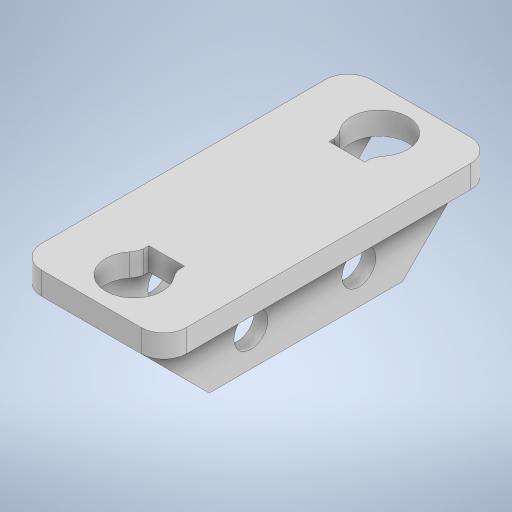
# Autodesk Inventor part: Magnet Mount
Saved by Autodesk Inventor 2023.1 (Build 271208000, 208)
## iProperties
Created: 2022-11-07
Part Number: Magnet Mount
Material: Generic
Document SubType Name: Modeling
Designer: nicol
Density: 1 g/cm^3
Appearance: Default
Author: nicol
Autodesk Inventor part; units mm, degrees
ref_plane "YZ Plane" through (0, 0, 0) normal (1, 0, 0) x (0, 1, 0)
ref_plane "XZ Plane" through (0, 0, 0) normal (0, 1, 0) x (-1, 0, 0)
ref_plane "XY Plane" through (0, 0, 0) normal (0, 0, 1) x (1, 0, 0)
sketch "Sketch1" plane through (0, 0, 0) normal (0, 1, 0) x (-1, 0, 0)
  line L0 (0, 0) -> (6.38, 0)
  line L1 (6.38, 0) -> (6.38, -20.1)
  line L2 (6.38, -20.1) -> (0, -20.1)
  line L3 (0, -20.1) -> (0, 0)
  line L4 (4.68, -1.7) -> (1.56, -1.7)
  line L5 (1.56, -1.7) -> (1.56, -2.17)
  line L6 (1.56, -2.17) -> (4.68, -2.17)
  line L7 (4.68, -2.17) -> (4.68, -1.7)
  line L8 (4.68, -18.03) -> (1.56, -18.03)
  line L9 (1.56, -18.03) -> (1.56, -18.5)
  line L10 (1.56, -18.5) -> (4.68, -18.5)
  line L11 (4.68, -18.5) -> (4.68, -18.03)
  line L12 (7.58, 4.4) -> (-1.2, 4.4)
  line L13 (-1.2, 4.4) -> (-1.2, -24.6)
  line L14 (-1.2, -24.6) -> (7.58, -24.6)
  line L15 (7.58, -24.6) -> (7.58, 4.4)
  circle A0 centre (3.12, -20.9) radius 2.5
  circle A1 centre (3.12, 0.7) radius 2.5
  line L16 (5.105, 3.2) -> (1.56, 3.2) construction
  line L17 (5.6212, -23.4) -> (1.5588, -23.4) construction
  point P0 (3.12, -18.5)
  point P1 (3.82, -1.7)
  point P2 (2.42, -18.5)
  point P3 (2.42, -1.7)
  point P4 (3.82, -18.5)
  dimension "d0" = 20.1
  dimension "d1" = 6.38
  dimension "d2" = 0.47
  dimension "d3" = 3.12
  dimension "d4" = 1.7
  dimension "d5" = 1.7
  dimension "d6" = 1.6
  dimension "d7" = 1.7
  dimension "d8" = 5
  dimension "d9" = 1.2
  dimension "d10" = 1.2
  dimension "d11" = 1.2
  dimension "d12" = 1.2
  dimension "d15" = 2.4
  dimension "d16" = 2.4
  constraints: 36 end point, 8 parallel, 6 horizontal, 4 perpendicular, 2 centre point, 2 equal length, 2 tangent, 2 vertical alignment, 1 equal radius, 1 midpoint
  measures "d0" distance of L0.end L1.end
  measures "d1" distance of L0.start L0.end
  measures "d2" distance of L6.end L4.start
  measures "d3" distance of L5.end L6.end
  measures "d4" distance between parallel lines of L1 L7
  measures "d5" distance between parallel lines of L0 L4
  measures "d6" distance between parallel lines of L2 L10
  measures "d7" distance between parallel lines of L1 L11
  measures "d8" diameter of A0
  measures "d9" distance between parallel lines of L13 L3
  measures "d10" distance between parallel lines of L15 L1
  measures "d11" distance between parallel lines of L12 L16
  measures "d12" distance between parallel lines of L14 L17
  measures "d15" distance from line of A0.centre L10
  measures "d16" distance from line of L4 A1.centre
extrude "Extrusion1" add sketch "Sketch1" along normal blind 2 contours L0 A1 L4 L5 L6 L7 L1 L2 A0 L10 L11 L8 L9 L3 | L15 L14 L13 L12
fillet "Fillet1" radius 2 4 edges at (-3.82, 1, -1.7) (-2.42, 1, -1.7) (-2.42, 1, -18.5) (-3.82, 1, -18.5)
sketch "Sketch2" plane through (0, 0, 0) normal (0, -1, 0) x (1, 0, 0)
  line L0 (1.2, 4.4) -> (1.2, -24.6) projected
  line L1 (1.2, 4.4) -> (0, 4.4)
  line L2 (0, 4.4) -> (0, -24.6)
  line L3 (0, -24.6) -> (1.2, -24.6)
  line L4 (1.2, -24.6) -> (1.2, 4.4)
  line L5 (1.2, -24.6) -> (-7.58, -24.6) projected
  line L6 (-7.58, -24.6) -> (-7.58, 4.4) projected
  line L7 (-7.58, 4.4) -> (-6.38, 4.4)
  line L8 (-6.38, 4.4) -> (-6.38, -24.6)
  line L9 (-6.38, -24.6) -> (-7.58, -24.6)
  line L10 (-7.58, -24.6) -> (-7.58, 4.4)
  point P0 (0, 0)
  dimension "d18" = 1.2
  dimension "d19" = 1.2
  constraints: 16 end point, 4 parallel, 2 collinear, 2 horizontal, 2 perpendicular
  measures "d18" distance between parallel lines of L0 L2
  measures "d19" distance of L8.end L9.end
extrude "Extrusion2" add sketch "Sketch2" along normal blind 6
sketch "Sketch3" plane through (1.2, 2, -24.6) normal (0, 0, -1) x (-1, 0, 0)
  line L0 (1.2, -2) -> (7.58, -2) projected
  line L1 (7.58, -2) -> (7.58, -8) projected
  line L2 (8.78, -8) -> (7.58, -8) projected
  line L3 (8.78, -8) -> (8.78, 0) projected
  line L4 (0, 0) -> (8.78, 0) projected
  line L5 (0, -8) -> (0, 0) projected
  line L6 (1.2, -8) -> (0, -8) projected
  line L7 (1.2, -2) -> (1.2, -8) projected
  line L8 (-2, -2) -> (10.78, -2)
  line L9 (10.78, -2) -> (10.78, 0)
  line L10 (10.78, 0) -> (-2, 0)
  line L11 (-2, 0) -> (-2, -2)
  line L12 (1.2, -2) -> (7.58, -2) projected
  line L13 (0, 0) -> (8.78, 0) projected
  point P0 (8.78, 0)
  point P1 (8.78, -2)
  point P2 (0, -2)
  dimension "d22" = 2
  dimension "d23" = 2
  constraints: 8 end point, 2 collinear, 2 parallel, 1 horizontal, 1 perpendicular
  measures "d22" distance between parallel lines of L11 L5
  measures "d23" distance between parallel lines of L9 L3
extrude "Extrusion3" add sketch "Sketch3" against normal up to surface (29 mm away) contours L8 L11 L10 L5 | L3 L10 L9 L8
sketch "Sketch4" plane through (-7.58, -6, -24.6) normal (-1, 0, 0) x (0, 0, 1)
  line L0 (6.1, 6) -> (6.57, 6) projected
  line L1 (6.57, 6) -> (6.57, 8) projected
  line L2 (6.1, 8) -> (6.57, 8) projected
  line L3 (6.1, 6) -> (6.1, 8) projected
  line L4 (22.43, 6) -> (22.9, 6) projected
  line L5 (22.9, 6) -> (22.9, 8) projected
  line L6 (22.43, 8) -> (22.9, 8) projected
  line L7 (22.43, 6) -> (22.43, 8) projected
  line L8 (29, 6) -> (0, 6) projected
  point P0 (24.6, 6)
  point P1 (9.8342, 3)
  point P2 (19.3342, 3)
  dimension "d26" = 9.5
  dimension "d27" = 3
  constraints: 1 horizontal alignment
  measures "d26" distance of point (19.334, 3) point (9.834, 3)
  measures "d27" distance from line of L8 point (9.834, 3)
hole "Hole1" at (-7.58, -3, -14.7658) at (-7.58, -3, -5.2658) direction (1, 0, 0) diameter 3 end through all
fillet "Fillet2" radius 2 4 edges at (-9.58, 1, -24.6) (-9.58, 1, 4.4) (3.2, 1, -24.6) (3.2, 1, 4.4)
chamfer "Chamfer1" distance 6 angle 45 4 edges at (0.6, -6, -24.6) (0.6, -6, 4.4) (-6.98, -6, 4.4) (-6.98, -6, -24.6)
equation "\"d10\" = d9"
equation "\"d11\" = d9"
body "Solid1"
